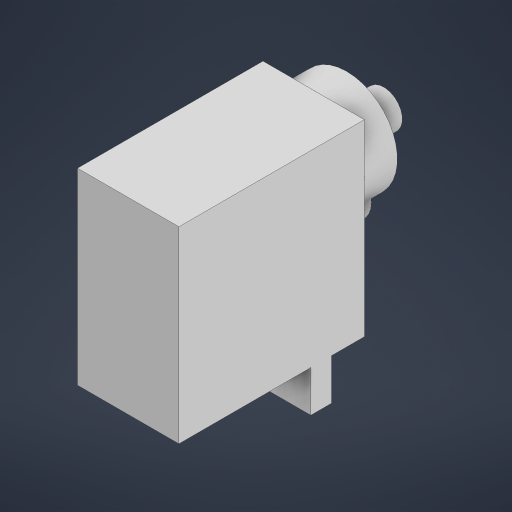
# Autodesk Inventor part: Motor
Saved by Autodesk Inventor 2024.2 (Build 282272000, 272)
## iProperties
Created: 2024-02-24
Part Number: Motor
Material: Generisch
Document SubType Name: Modeling
Designer: jacob
Density: 1 g/cm^3
Appearance: Vorgabe
Author: jacob
Autodesk Inventor part; units mm, degrees
ref_plane "YZ Plane" through (0, 0, 0) normal (1, 0, 0) x (0, 1, 0)
ref_plane "XZ Plane" through (0, 0, 0) normal (0, 1, 0) x (-1, 0, 0)
ref_plane "XY Plane" through (0, 0, 0) normal (0, 0, 1) x (1, 0, 0)
sketch "Skizze1" plane through (0, 0, 0) normal (1, 0, 0) x (0, 1, 0)
  line L0 (11.4, 22.5) -> (11.4, 6.5)
  line L1 (11.4, 6.5) -> (16.4, 6.5)
  line L2 (16.4, 6.5) -> (16.4, 4)
  line L3 (16.4, 4) -> (11.4, 4)
  line L4 (11.4, 4) -> (11.4, 0)
  line L5 (11.4, 0) -> (0, 0)
  line L6 (0, 0) -> (0, 22.5)
  line L7 (0, 22.5) -> (11.4, 22.5)
  dimension "d0" = 2.5
  dimension "d1" = 5
  dimension "d2" = 4
  dimension "d3" = 16
  dimension "d4" = 11.4
  constraints: 16 end point, 6 perpendicular, 2 point on line, 1 coincident, 1 vertical
  measures "d0" distance of L1.end L2.end
  measures "d1" distance of L2.end L3.end
  measures "d2" distance of L3.end L4.end
  measures "d3" distance of L0.start L0.end
  measures "d4" distance of L6.end L0.start
extrude "Extrusion1" add sketch "Skizze1" along normal blind 12.3
mirror "Spiegeln1" about plane through (0, 0, 22.5) normal (0, -1, 0) of "Extrusion1"
sketch "Skizze2" plane through (12.3, 11.4, 0) normal (0, 0, -1) x (-1, 0, 0)
  circle A0 centre (6.15, -6.15) radius 6.15
  line L0 (12.3, 0) -> (0, 0) projected
  line L1 (6.15, 0) -> (6.15, -6.15) construction
  line L2 (6.15, -6.15) -> (12.3, -6.15) construction
  line L3 (12.3, 0) -> (12.3, -22.8) construction
  point P0 (12.3, -11.4)
  constraints: 4 end point, 2 perpendicular, 1 centre point, 1 midpoint, 1 point on line, 1 tangent, 1 vertical, 1 vertical alignment
extrude "Extrusion2" add sketch "Skizze2" along normal blind 4
sketch "Skizze3" plane through (6.15, 5.25, -4) normal (0, 0, -1) x (-1, 0, 0)
  arc A0 (-6.15, 0) -> (6.15, 0) centre (0, 0) ccw projected
  arc A1 (-2.9094, -5.4183) -> (2.9094, -5.4183) centre (0, -6.15) ccw
  point P0 (6.15, -5.25)
  dimension "d9" = 6
  constraints: 5 point on circle, 1 centre point, 1 vertical alignment
  measures "d9" diameter of A1
extrude "Extrusion3" add sketch "Skizze3" against normal up to surface (4 mm away)
sketch "Skizze4" plane through (0, 11.4, 4) normal (0, 0, -1) x (-1, 0, 0)
  line L0 (-12.3, -22.8) -> (-12.3, -27.8) projected
  line L1 (-12.3, 0) -> (-12.3, 5) projected
  line L2 (0, 5) -> (-12.3, 5) projected
  point P0 (0, -11.4)
  point P1 (-6.15, 2.5)
  point P2 (-6.15, -25.3)
  point P3 (-12.3, -25.3)
  point P4 (-12.3, 2.5)
  point P5 (-6.15, 5)
  constraints: 3 midpoint, 2 horizontal alignment, 2 vertical alignment
hole "Bohrung1" at (6.15, 13.9, 4) at (6.15, -13.9, 4) direction (0, 0, 1) diameter 3 end through all
sketch "Skizze5" plane through (12.3, 11.4, -4) normal (0, 0, -1) x (-1, 0, 0)
  circle A0 centre (6.15, -6.15) radius 2.25
  arc A1 (9.0594, -11.5683) -> (3.2406, -11.5683) centre (6.15, -6.15) ccw projected
  point P0 (12.3, -11.4)
  dimension "d19" = 4.5
  constraints: 1 centre point, 1 concentric
  measures "d19" diameter of A0
extrude "Extrusion4" add sketch "Skizze5" along normal blind 4.5
sketch "Skizze6" plane through (0, 0, 0) normal (-1, 0, 0) x (0, 0, 1)
  line L0 (6.5, 11.4) -> (22.5, 11.4) projected
  line L1 (4, 16.4) -> (6.5, 16.4)
  line L2 (6.5, 16.4) -> (6.5, 11.4)
  line L3 (6.5, 11.4) -> (4, 11.4)
  line L4 (4, 11.4) -> (4, 16.4)
  point P0 (0, 0)
  constraints: 8 end point, 2 parallel, 1 coincident, 1 horizontal, 1 perpendicular
extrude "Extrusion5" cut sketch "Skizze6" against normal through all
